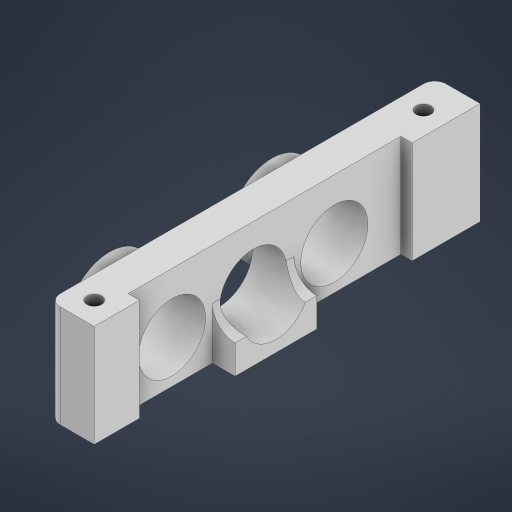
# Autodesk Inventor part: MotorMount_New
Saved by Autodesk Inventor 2023 (Build 270158000, 158)
## iProperties
Created: 2022-10-13
Part Number: MotorMount_New
Material: 一般
Document SubType Name: Modeling
Designer: neko2
Density: 1 g/cm^3
Appearance: 既定
Author: neko2
Autodesk Inventor part; units mm, degrees
ref_plane "YZ Plane" through (0, 0, 0) normal (1, 0, 0) x (0, 1, 0)
ref_plane "XZ Plane" through (0, 0, 0) normal (0, 1, 0) x (-1, 0, 0)
ref_plane "XY Plane" through (0, 0, 0) normal (0, 0, 1) x (1, 0, 0)
sketch "スケッチ1" plane through (0, 0, 0) normal (0, 1, 0) x (-1, 0, 0)
  line L0 (0, 0) -> (4, 0)
  line L1 (4, 0) -> (4, 34)
  line L2 (4, 34) -> (0, 34)
  line L3 (0, 34) -> (0, 30)
  line L4 (0, 30) -> (1, 30)
  line L5 (1, 30) -> (1, 6)
  line L6 (1, 6) -> (0, 6)
  line L7 (0, 6) -> (0, 0)
  dimension "d0" = 34
  dimension "d3" = 6
  dimension "d4" = 4
  dimension "d38" = 4
  dimension "d39" = 1
  constraints: 16 end point, 7 perpendicular, 1 horizontal, 1 point on line
  measures "d0" distance between parallel lines of L0 L2
  measures "d3" distance of L6.end L0.start
  measures "d4" distance of L2.end L3.end
  measures "d38" distance of L0.start L0.end
  measures "d39" distance of L5.end L6.end
extrude "押し出し1" add sketch "スケッチ1" along normal blind 9
sketch "スケッチ2" plane through (0, 9, 0) normal (0, 1, 0) x (1, 0, 0)
  circle A0 centre (-2, -3) radius 0.65
  circle A1 centre (-2, -32) radius 0.65
  line L0 (-4, -34) -> (0, -34) projected
  line L1 (-4, 0) -> (-4, -34) projected
  dimension "d7" = 1.3
  dimension "d10" = 29
  dimension "d27" = 2
  dimension "d40" = 2
  constraints: 2 centre point, 1 equal radius, 1 vertical alignment
  measures "d7" diameter of A0
  measures "d10" distance of A1.centre A0.centre
  measures "d27" distance from line of A1.centre L0
  measures "d40" distance from line of A1.centre L1
extrude "押し出し2" cut sketch "スケッチ2" against normal through all
sketch "スケッチ3" plane through (-1, 0, 30) normal (1, 0, 0) x (0, 0, -1)
  circle A0 centre (11, 3.95) radius 2.95
  line L0 (30, 0) -> (30, 9) projected
  line L1 (7.0914, 1) -> (14.9086, 1)
  line L2 (0, 0) -> (24, 0) projected
  circle A1 centre (3.8528, 3.75) radius 2.95
  line L3 (11, 3.95) -> (11, 0)
  line L4 (-0.0876, 0.8) -> (7.7932, 0.8)
  circle A2 centre (18.1472, 3.75) radius 2.95
  line L5 (-4, 0) -> (-4, 9) projected
  point P0 (11, 1)
  point P1 (3.8528, 0.8)
  dimension "d13" = 5.9
  dimension "d15" = 1
  dimension "d16" = 5.9
  dimension "d17" = 7.15
  dimension "d18" = 0.8
  dimension "d41" = 15
  constraints: 6 end point, 3 centre point, 2 horizontal, 2 midpoint, 2 tangent, 2 vertical alignment, 1 perpendicular, 1 point on line, 1 symmetric about line, 1 other
  measures "d13" diameter of A0
  measures "d15" distance between parallel lines of L2 L1
  measures "d16" diameter of A1
  measures "d17" distance of A1.centre L3.start
  measures "d18" distance between parallel lines of L2 L4
  measures "d41" distance from line of L5 L3.start
extrude "押し出し3" cut sketch "スケッチ3" against normal through all
sketch "スケッチ4" plane through (-4, 0, 68) normal (-1, 0, 0) x (0, 0, 1)
  line L0 (-68, 0) -> (-34, 0) projected
  line L1 (-68, 0) -> (-68, 9) projected
  line L2 (-68, 9) -> (-34, 9) projected
  line L3 (-34, 0) -> (-34, 9) projected
  circle A0 centre (-41.8528, 3.75) radius 3.75
  line L4 (-38, 0) -> (-62, 0) projected
  circle A1 centre (-56.1472, 3.75) radius 3.75
  circle A2 centre (-41.8528, 3.75) radius 2.95 projected
  circle A3 centre (-56.1472, 3.75) radius 2.95 projected
  circle A4 centre (-49, 3.95) radius 2.95 projected
  line L5 (-68, 0) -> (-34, 0) projected
  line L6 (-34, 0) -> (-34, 9) projected
  line L7 (-68, 9) -> (-34, 9) projected
  line L8 (-68, 0) -> (-68, 9) projected
  constraints: 2 centre point, 2 coincident, 2 tangent
extrude "押し出し4" add sketch "スケッチ4" along normal blind 2.5 contours A1 | A0
sketch "スケッチ5" plane through (-1, 0, 6) normal (1, 0, 0) x (0, 0, -1)
  line L0 (-24, 0) -> (0, 0) projected
  line L1 (-24, 0) -> (-24, 9) projected
  line L2 (-24, 9) -> (0, 9) projected
  line L3 (0, 0) -> (0, 9) projected
  circle A0 centre (-20.1472, 3.75) radius 3.75
  circle A1 centre (-5.8528, 3.75) radius 3.75
  line L4 (-16.5953, 2.5474) -> (-16.5953, 0)
  line L5 (-28, 0) -> (6, 0) projected
  line L6 (-16.5953, 2.5474) -> (-15.5953, 2.5474)
  line L7 (-9.4047, 2.5474) -> (-10.4047, 2.5474)
  line L8 (-9.4047, 2.5474) -> (-9.4047, 0)
  circle A2 centre (-20.1472, 3.75) radius 2.95 projected
  circle A3 centre (-5.8528, 3.75) radius 2.95 projected
  circle A4 centre (-13, 3.95) radius 2.95 projected
  line L9 (-24, 0) -> (0, 0) projected
  line L10 (0, 0) -> (0, 9) projected
  line L11 (-24, 9) -> (0, 9) projected
  line L12 (-24, 0) -> (-24, 9) projected
  circle A5 centre (-20.1472, 3.75) radius 2.95 projected
  circle A6 centre (-5.8528, 3.75) radius 2.95 projected
  circle A7 centre (-13, 3.95) radius 2.95 projected
  point P0 (-20.1472, 0)
  point P1 (-5.8528, 0)
  dimension "d31" = 7.5
  dimension "d32" = 1
  constraints: 8 end point, 5 point on line, 3 perpendicular, 1 point on circle, 10 other
  measures "d32" distance of L4.start L6.end
extrude "押し出し5" add sketch "スケッチ5" along normal blind 2 contours L4 L6 A4 L7 L8 L0
fillet "フィレット1" radius 2 2 edges at (-1, 2.5474, 22.0953) (-1, 2.5474, 15.9047)
fillet "フィレット2" radius 1 2 edges at (-4, 4.5, 0) (-4, 4.5, 34)
fillet "フィレット3" radius 0.5 4 edges at (-4, 6.4017, 23.4956) (-4, 1.0983, 28.7989) (-4, 6.4017, 9.2011) (-4, 1.0983, 14.5044)
